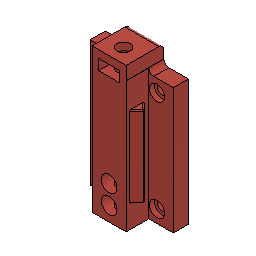
01 Laser Mount v1 (Autodesk Fusion 360 design; units mm, degrees)
Autodesk Fusion 360 part; units mm, degrees
sketch "Sketch1" plane through (0, 0, 0) normal (0, 1, 0) x (1, 0, 0)
  line L0 (-6.75, 9) -> (-16.5, 9)
  line L1 (16.5, 9) -> (6.75, 9)
  line L2 (6.75, 9) -> (6.75, 7.142)
  line L3 (6.75, 7.142) -> (9.4695, 4.4264)
  arc A0 (9.4698, 4.0728) -> (9.4695, 4.4264) centre (9.2929, 4.2495) ccw
  line L4 (9.4698, 4.0728) -> (6.75, 1.3491)
  line L5 (6.75, 1.3491) -> (6.75, 0)
  line L6 (6.75, 0) -> (-6.75, 0)
  line L7 (-6.75, 0) -> (-6.75, 1.3491)
  line L8 (-6.75, 1.3491) -> (-9.4698, 4.0728)
  arc A1 (-9.4695, 4.4264) -> (-9.4698, 4.0728) centre (-9.2929, 4.2495) ccw
  line L9 (-9.4695, 4.4264) -> (-6.75, 7.142)
  line L10 (-6.75, 7.142) -> (-6.75, 9)
  line L11 (0, 0) -> (0, 15.75)
  line L12 (-16.5, 9) -> (-16.5, 15)
  line L13 (-16.5, 15) -> (16.5, 15)
  line L14 (16.5, 15) -> (16.5, 9)
  dimension "d2" = 33
  dimension "d3" = 16.5
  dimension "d4" = 6
  constraint tangent L3 A0
  constraint tangent A0 L4
  constraint tangent L8 A1
  constraint tangent A1 L9
  constraint midpoint L6 L11.start
  constraint perpendicular L6 L11
  constraint perpendicular L0 L12
  constraint perpendicular L12 L13
  constraint perpendicular L1 L14
  measures "d2" distance of L12.end L13.end
  measures "d3" distance of L11 L12
  measures "d4" distance of L0.end L12.end
extrude "Extrude1" add sketch "Sketch1" along normal blind 50
sketch "Sketch2" plane through (0, 0, -15) normal (0, 0, -1) x (-1, 0, 0)
  line L0 (-16.5, 0) -> (16.5, 0)
  line L1 (16.5, 0) -> (16.5, 50)
  line L2 (16.5, 50) -> (-16.5, 50)
  line L3 (-16.5, 50) -> (-16.5, 0)
  line L4 (0, 50) -> (0, 0)
  circle A0 centre (-10, 45) radius 1.75
  line L5 (0, 25) -> (-16.5, 25)
  circle A1 centre (10, 45) radius 1.75
  circle A2 centre (-10, 5) radius 1.75
  circle A3 centre (10, 5) radius 1.75
  circle A4 centre (0, 13.25) radius 1.75
  circle A5 centre (0, 5.75) radius 1.75
  dimension "d7" = 3.5
  dimension "d8" = 10
  dimension "d10" = 20
  dimension "d63" = 3.5
  dimension "d64" = 31.75
  dimension "d65" = 3.5
  dimension "d66" = 7.5
  constraint midpoint L2 L4.start
  constraint coincident L4.end origin
  constraint midpoint L4 L5.start
  constraint midpoint L3 L5.end
  constraint symmetric L4 A0 A1
  constraint symmetric A0 L5 A2
  constraint symmetric L5 A1 A3
  constraint coincident L4 A4.centre
  constraint coincident L4 A5.centre
  measures "d7" diameter of A0
  measures "d8" distance of L4 A0.centre
  measures "d10" distance of A0.centre L5
  measures "d63" diameter of A4
  measures "d64" vertical distance of A0.centre A4.centre
  measures "d65" diameter of A5
  measures "d66" distance of A4.centre A5.centre
extrude "Extrude2" cut sketch "Sketch2" against normal through all contours A0 | A1 | A2 | A3
sketch "Sketch3" plane through (0, 0, -9) normal (0, 0, 1) x (1, 0, 0)
  line L0 (-6.75, 50) -> (-16.5, 50)
  line L1 (-16.5, 50) -> (-16.5, 0)
  line L2 (-16.5, 0) -> (-6.75, 0)
  line L3 (-6.75, 0) -> (-6.75, 50)
  circle A0 centre (-10, 45) radius 3
  circle A1 centre (10, 45) radius 3
  circle A2 centre (10, 45) radius 1.75
  circle A3 centre (-10, 5) radius 3
  circle A4 centre (10, 5) radius 3
  circle A5 centre (-10, 45) radius 1.75
  circle A6 centre (-10, 5) radius 1.75
  dimension "d12" = 6
  dimension "d13" = 6
  dimension "d14" = 6
  dimension "d15" = 6
  dimension "d67" = 20
  constraint concentric A0 A5
  constraint concentric A1 A2
  constraint concentric A3 A6
  measures "d12" diameter of A0
  measures "d13" diameter of A1
  measures "d14" diameter of A3
  measures "d15" diameter of A4
  measures "d67" distance of A3.centre A4.centre
extrude "Extrude4" cut sketch "Sketch3" along normal blind 20 and the other way blind 2 contours A0 | A1 | A2 | A3 | A4 | A5 | A6
sketch "Sketch4" plane through (0, 50, 0) normal (0, 1, 0) x (-1, 0, 0)
  arc A0 (9.4695, -4.4264) -> (9.4698, -4.0728) centre (9.2929, -4.2495) ccw
  line L0 (9.4698, -4.0728) -> (6.75, -1.3491)
  line L1 (6.75, -1.3491) -> (6.75, 0)
  line L2 (6.75, 0) -> (-6.75, 0)
  line L3 (-6.75, 0) -> (-6.75, -1.3491)
  line L4 (-6.75, -1.3491) -> (-9.4698, -4.0728)
  arc A1 (-9.4698, -4.0728) -> (-9.4695, -4.4264) centre (-9.2929, -4.2495) ccw
  line L5 (-9.4695, -4.4264) -> (-6.75, -7.142)
  line L6 (-6.75, -7.142) -> (-6.75, -9)
  line L7 (-6.75, -9) -> (-16.5, -9)
  line L8 (-16.5, -9) -> (-16.5, -15)
  line L9 (-16.5, -15) -> (16.5, -15)
  line L10 (16.5, -15) -> (16.5, -9)
  line L11 (16.5, -9) -> (6.75, -9)
  line L12 (6.75, -9) -> (6.75, -7.142)
  line L13 (6.75, -7.142) -> (9.4695, -4.4264)
  line L14 (6.75, 0) -> (-6.75, 0)
  line L15 (6.75, -15) -> (6.75, 0)
  line L16 (6.75, -15) -> (-6.7448, -15)
  line L17 (-6.75, 0) -> (-6.7448, -15)
  constraint horizontal L14
  constraint vertical L15
  constraint coincident L1.end L2.start
  constraint coincident L9 L15.start
  constraint coincident L9 L16.end
sketch "Sketch5" plane through (0, 0, 0) normal (0, -1, 0) x (1, 0, 0)
  arc A0 (-9.4698, -4.0728) -> (-9.4695, -4.4264) centre (-9.2929, -4.2495) ccw
  line L0 (-9.4695, -4.4264) -> (-6.75, -7.142)
  line L1 (-6.75, -7.142) -> (-6.75, -9)
  line L2 (-6.75, -9) -> (-16.5, -9)
  line L3 (-16.5, -9) -> (-16.5, -15)
  line L4 (-16.5, -15) -> (16.5, -15)
  line L5 (16.5, -15) -> (16.5, -9)
  line L6 (16.5, -9) -> (6.75, -9)
  line L7 (6.75, -9) -> (6.75, -7.142)
  line L8 (6.75, -7.142) -> (9.4695, -4.4264)
  arc A1 (9.4695, -4.4264) -> (9.4698, -4.0728) centre (9.2929, -4.2495) ccw
  line L9 (9.4698, -4.0728) -> (6.75, -1.3491)
  line L10 (6.75, -1.3491) -> (6.75, 0)
  line L11 (6.75, 0) -> (-6.75, 0)
  line L12 (-6.75, 0) -> (-6.75, -1.3491)
  line L13 (-6.75, -1.3491) -> (-9.4698, -4.0728)
  line L14 (-6.75, 0) -> (-16.5, 0)
  line L15 (-16.5, 0) -> (-16.5, -9)
  line L16 (-16.5, -9) -> (-6.75, -9)
  line L17 (-6.75, -9) -> (-6.75, 0)
  line L18 (6.75, 0) -> (16.5, 0)
  line L19 (16.5, 0) -> (16.5, -9)
  line L20 (16.5, -9) -> (6.75, -9)
  line L21 (6.75, -9) -> (6.75, 0)
  constraint horizontal L14
  constraint vertical L15
  constraint horizontal L16
  constraint vertical L17
  constraint coincident L2.end L3.start
  constraint coincident L11.end L12.start
  constraint horizontal L18
  constraint vertical L19
  constraint horizontal L20
  constraint vertical L21
  constraint coincident L5.end L6.start
  constraint coincident L10.end L11.start
extrude "Extrude6" cut sketch "Sketch5" against normal blind 9 contours A0 L0 L13 L17 | A0 L0 L1 L2 L12 L13 L14 L15 L16 L17 | L6 L7 L8 A1 L9 L10 L18 L19 L20 L21 | L8 A1 L9 L21
extrude "Extrude9" add sketch "Sketch4" along normal blind 4.25 contours L1 L2 L3 L9 L12 L14 L15 L16 L17
sketch "Sketch11" plane through (0, 54.25, 0) normal (0, 1, 0) x (-1, 0, 0)
  line L0 (6.75, -15) -> (6.75, 0)
  line L1 (6.75, 0) -> (-6.75, 0)
  line L2 (-6.75, 0) -> (-6.7448, -15)
  line L3 (-6.7448, -15) -> (6.75, -15)
  circle A0 centre (0, -5.75) radius 2.625
  dimension "d37" = 5.25
  dimension "d38" = 5.75
  measures "d37" diameter of A0
  measures "d38" distance of origin A0.centre
extrude "Extrude10" cut sketch "Sketch11" against normal through all contours A0
sketch "Sketch12" plane through (0, 54.25, 0) normal (0, 1, 0) x (-1, 0, 0)
  circle A0 centre (0, -5.75) radius 2.625
  line L0 (6.75, -15) -> (6.75, 0)
  line L1 (6.75, 0) -> (-6.75, 0)
  line L2 (-6.75, 0) -> (-6.7448, -15)
  line L3 (-6.7448, -15) -> (6.75, -15)
  line L4 (-4.2, 0) -> (-4.2, -8.4249)
  line L5 (-4.2, -8.4249) -> (0, -10.8497)
  line L6 (0, -10.8497) -> (4.2, -8.4249)
  line L7 (4.2, -8.4249) -> (4.2, 0)
  line L8 (4.2, 0) -> (-4.2, 0)
  point P0 (0, -5.75)
  constraint coincident P0 A0.centre
  constraint coincident L1 L7.end
  constraint coincident L1 L4.start
  constraint perpendicular L4 L8
extrude "Extrude11" cut sketch "Sketch12" against normal up to surface (4.25 mm away) contours L1 L4 L5 L6 L7 L8
sketch "Sketch13" plane through (0, 54.25, 0) normal (0, 1, 0) x (-1, 0, 0)
  line L0 (-4.2, -8.4249) -> (-4.2, 0)
  line L1 (-4.2, 0) -> (-6.75, 0)
  line L2 (-6.75, 0) -> (-6.7448, -15)
  line L3 (-6.7448, -15) -> (6.75, -15)
  line L4 (6.75, -15) -> (6.75, 0)
  line L5 (6.75, 0) -> (4.2, 0)
  line L6 (4.2, 0) -> (4.2, -8.4249)
  line L7 (4.2, -8.4249) -> (0, -10.8497)
  line L8 (0, -10.8497) -> (-4.2, -8.4249)
  line L9 (6.75, -15) -> (-6.75, -15)
  line L10 (-6.75, -15) -> (-6.75, 0)
  line L11 (-6.75, 0) -> (6.75, 0)
  line L12 (6.75, 0) -> (6.75, -15)
  constraint horizontal L9
  constraint vertical L10
  constraint horizontal L11
  constraint vertical L12
  constraint coincident L1.end L2.start
  constraint coincident L3.end L4.start
extrude "Extrude12" add sketch "Sketch13" along normal blind 3 contours L0 L1 L2 L3 L4 L5 L6 L7 L8 L9 L11 L12 | L0 L6 L7 L8 L11
sketch "Sketch14" plane through (0, 57.25, 0) normal (0, 1, 0) x (-1, 0, 0)
  line L0 (-6.75, 0) -> (-6.7448, -15)
  line L1 (-6.7448, -15) -> (6.75, -15)
  line L2 (6.75, -15) -> (6.75, 0)
  line L3 (6.75, 0) -> (-6.75, 0)
  circle A0 centre (0, -5.75) radius 2.625
  circle A1 centre (0, -5.75) radius 2.625
  constraint concentric A0 A1
extrude "Extrude13" cut sketch "Sketch14" against normal blind 3 contours A0 A1
sketch "Sketch15" plane through (0, 57.25, 0) normal (0, 1, 0) x (-1, 0, 0)
  circle A0 centre (0, -5.75) radius 2.625
  line L0 (-6.75, 0) -> (-6.7448, -15)
  line L1 (-6.7448, -15) -> (6.75, -15)
  line L2 (6.75, -15) -> (6.75, 0)
  line L3 (6.75, 0) -> (-6.75, 0)
  line L4 (16.5, -9) -> (6.75, -9)
  line L5 (6.75, -9) -> (6.75, 0)
  line L6 (6.75, 0) -> (16.5, 0)
  line L7 (16.5, 0) -> (16.5, -9)
  line L8 (-16.5, -9) -> (-6.75, -9)
  line L9 (-6.75, -9) -> (-6.75, 0)
  line L10 (-6.75, 0) -> (-16.5, 0)
  line L11 (-16.5, 0) -> (-16.5, -9)
  point P0 (16.5, -9)
  point P1 (-16.5, -9)
  constraint horizontal L4
  constraint vertical L5
  constraint horizontal L6
  constraint vertical L7
  constraint coincident L2.end L3.start
  constraint coincident P0 L4.start
  constraint horizontal L8
  constraint vertical L9
  constraint horizontal L10
  constraint vertical L11
  constraint coincident L0.start L3.end
  constraint coincident P1 L8.start
extrude "Extrude14" cut sketch "Sketch15" against normal blind 16 contours L8 L9 L10 L11 | L2 L4 L5 L6 L7
fillet "Fillet1" radius 2 1 edges at (-0.0026, 57.25, -15)
fillet "Fillet2" radius 2 1 edges at (6.7474, 50, -7.5)
fillet "Fillet3" radius 2 1 edges at (-6.75, 50, -12)
fillet "Fillet4" radius 0.5 3 edges at (-8.1099, 41.25, -2.7109) (-9.5429, 41.25, -4.2497) (-8.1098, 41.25, -5.7842)
fillet "Fillet5" radius 0.5 3 edges at (-8.1098, 9, -5.7842) (-9.5429, 9, -4.2497) (-8.1099, 9, -2.7109)
fillet "Fillet6" radius 0.5 3 edges at (8.1099, 9, -2.7109) (9.5429, 9, -4.2497) (8.1098, 9, -5.7842)
fillet "Fillet7" radius 0.5 3 edges at (8.1098, 41.25, -5.7842) (9.5429, 41.25, -4.2497) (8.1099, 41.25, -2.7109)
extrude "Extrude15" cut sketch "Sketch2" against normal up to surface (15 mm away) contours L4 A5 | L4 A5 | L4 A4 | L4 A4
sketch "Sketch16" plane through (0, 0, 0) normal (0, 0, 1) x (1, 0, 0)
  circle A0 centre (0, 13.25) radius 1.75
  circle A1 centre (0, 5.75) radius 1.75
  line L0 (4.2, 54.25) -> (4.2, 50)
  line L1 (4.2, 50) -> (-4.2, 50)
  line L2 (-4.2, 50) -> (-4.2, 54.25)
  line L3 (-4.2, 54.25) -> (4.2, 54.25)
  line L4 (6.75, 0) -> (6.75, 52)
  line L5 (6.75, 52) -> (6.75, 57.25)
  line L6 (6.75, 57.25) -> (-6.75, 57.25)
  line L7 (-6.75, 57.25) -> (-6.75, 0)
  line L8 (-6.75, 0) -> (6.75, 0)
  circle A2 centre (0, 13.25) radius 3.125
  circle A3 centre (0, 5.75) radius 3.125
  dimension "d70" = 6.25
  dimension "d71" = 6.25
  constraint concentric A0 A2
  constraint concentric A1 A3
  measures "d70" diameter of A2
  measures "d71" diameter of A3
extrude "Extrude16" cut sketch "Sketch16" against normal up to surface (11 mm away) contours A2 | A3
